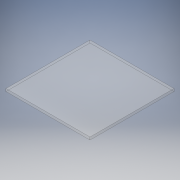
# Autodesk Inventor part: CollectorFloor
Saved by Autodesk Inventor 2019 (Build 230136000, 136)
## iProperties
Created: 2018-10-04
Part Number: CollectorFloor
Material: Polycarbonate, Clear
Document SubType Name: Modeling
Designer: User
Density: 1.2 g/cm^3
Appearance: Polycarbonate - Clear
Mass: 39.329 g
Surface Area: 219.354 cm^2
Volume: 32.7741 cm^3
Author: User
Autodesk Inventor part; units mm, degrees
ref_plane "YZ Plane" through (0, 0, 0) normal (1, 0, 0) x (0, 1, 0)
ref_plane "XZ Plane" through (0, 0, 0) normal (0, 1, 0) x (-1, 0, 0)
ref_plane "XY Plane" through (0, 0, 0) normal (0, 0, 1) x (1, 0, 0)
sketch "Sketch1" plane through (0, 0, 0) normal (0, 1, 0) x (-1, 0, 0)
  line L0 (0, 0) -> (101.6, 0)
  line L1 (101.6, 0) -> (101.6, -101.6)
  line L2 (101.6, -101.6) -> (0, -101.6)
  line L3 (0, -101.6) -> (0, 0)
  dimension "d0" = 101.6
  dimension "d1" = 101.6
  constraints: 8 end point, 2 parallel, 1 horizontal, 1 perpendicular
  measures "d0" distance of L1.end L2.end
  measures "d1" distance of L0.end L1.end
extrude "Extrusion1" add sketch "Sketch1" along normal blind 3.175
body "Solid1"
